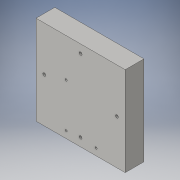
# Autodesk Inventor part: speakerbottom
Saved by Autodesk Inventor 2016 (Build 200138000, 138)
## iProperties
Created: 2018-09-28
Part Number: speakerbottom
Material: Generic
Document SubType Name: Modeling
Designer: student
Density: 1 g/cm^3
Appearance: Default
Author: student
Autodesk Inventor part; units mm, degrees
ref_plane "YZ Plane" through (0, 0, 0) normal (1, 0, 0) x (0, 1, 0)
ref_plane "XZ Plane" through (0, 0, 0) normal (0, 1, 0) x (-1, 0, 0)
ref_plane "XY Plane" through (0, 0, 0) normal (0, 0, 1) x (1, 0, 0)
sketch "Sketch1" plane through (0, 0, 0) normal (0, 0, 1) x (1, 0, 0)
  line L0 (0, 0) -> (120.65, 0)
  line L1 (120.65, 0) -> (120.65, 120.65)
  line L2 (120.65, 120.65) -> (0, 120.65)
  line L3 (0, 120.65) -> (0, 0)
  circle A0 centre (11.2141, 60.325) radius 1.9431
  circle A1 centre (60.325, 11.2141) radius 1.9431
  circle A2 centre (109.4359, 60.325) radius 1.9431
  circle A3 centre (60.325, 109.4359) radius 1.9431
  circle A4 centre (81.3054, 9.2329) radius 1.397
  circle A5 centre (40.7924, 9.2329) radius 1.397
  circle A6 centre (40.7924, 68.7451) radius 1.397
  point P0 (60.325, 60.325)
  dimension "d2" = 120.65
  dimension "d3" = 120.65
  dimension "d10" = 3.8862
  dimension "d13" = 360
  dimension "d33" = 2.794
  dimension "d35" = 2.794
  dimension "d37" = 2.794
  constraints: 8 end point, 7 centre point, 2 parallel, 1 horizontal, 1 perpendicular, 9 other
  measures "d2" distance of L2.end L1.end
  measures "d3" distance of L1.end L0.end
  measures "d10" diameter of A0
  measures "d33" diameter of A4
  measures "d35" diameter of A5
  measures "d37" diameter of A6
extrude "Extrusion4" add sketch "Sketch1" along normal blind 25.4
body "Solid4"
